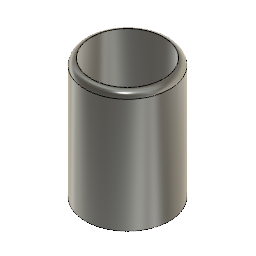
vase tema lab1 (Autodesk Fusion 360 design; units mm, degrees)
Autodesk Fusion 360 part; units mm, degrees
sketch "Sketch1" plane through (0, 0, 0) normal (0, 0, 1) x (1, 0, 0)
  circle A0 centre (0, 0) radius 35
  dimension "d6" = 70
  constraint coincident A0.centre origin
  measures "d6" diameter of A0
extrude "Extrude1" add sketch "Sketch1" along normal blind 100
sketch "Sketch2" plane through (0, 0, 100) normal (0, 0, 1) x (-1, 0, 0)
  circle A0 centre (0, 0) radius 35
  circle A1 centre (0, 0) radius 29.9384
  constraint coincident A0.centre A1.centre
extrude "Extrude2" cut sketch "Sketch2" against normal blind 55 contours A1
fillet "Fillet1" radius 5 1 edges at (-32.6315, -12.6565, 100)
